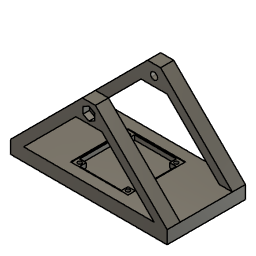
Pitch Control Base v3 (Autodesk Fusion 360 design; units mm, degrees)
Autodesk Fusion 360 part; units mm, degrees
note: some values were not read from the file. Set by a fixed rule: which sketch regions a step uses.
sketch "Sketch1" plane through (0, 0, 0) normal (0, 1, 0) x (1, 0, 0)
  line L0 (60, -30) -> (-60, -30)
  line L1 (-60, -30) -> (-60, 30)
  line L2 (-60, 30) -> (60, 30)
  line L3 (60, 30) -> (60, -30)
  line L4 (60, -30) -> (-60, 30) construction
  line L5 (-60, -30) -> (60, 30) construction
  constraint horizontal L0
  constraint perpendicular L0 L1
  constraint parallel L0 L2
  constraint parallel L1 L3
  constraint coincident L4 origin
  constraint coincident L5 origin
extrude "Extrude1" add sketch "Sketch1" along normal blind 10
sketch "Sketch2" plane through (0, 0, 0) normal (0, 0, 1) x (1, 0, 0)
  line L0 (-60, 10) -> (-5, 65)
  line L1 (-5, 65) -> (5, 65)
  line L2 (5, 65) -> (60, 10)
  line L3 (60, 10) -> (50, 10)
  line L4 (-50, 10) -> (-60, 10)
  line L5 (-50, 10) -> (-10, 50)
  line L6 (-10, 50) -> (10, 50)
  line L7 (10, 50) -> (50, 10)
  constraint horizontal L1
  constraint parallel L1 L3
  constraint horizontal L4
  constraint parallel L0 L5
  constraint parallel L4 L6
extrude "Extrude2" add sketch "Sketch2" along normal mid plane 60
sketch "Sketch3" plane through (0, 0, 30) normal (0, 0, 1) x (1, 0, 0)
  line L0 (50, 10) -> (-50, 10)
  line L1 (-50, 10) -> (-10, 50)
  line L2 (-10, 50) -> (10, 50)
  line L3 (10, 50) -> (50, 10)
  line L4 (60, 10) -> (5, 65)
  line L5 (5, 65) -> (-5, 65)
  line L6 (-5, 65) -> (-60, 10)
  line L7 (-60, 10) -> (-60, 0)
  line L8 (-60, 0) -> (60, 0)
  line L9 (60, 0) -> (60, 10)
  line L10 (0, 62) -> (4.5, 59.5)
  line L11 (4.5, 59.5) -> (4.5, 54.5)
  line L12 (4.5, 54.5) -> (0, 52)
  line L13 (0, 52) -> (-4.5, 54.5)
  line L14 (-4.5, 54.5) -> (-4.5, 59.5)
  line L15 (-4.5, 59.5) -> (0, 62)
  circle A0 centre (0, 57) radius 2.7
  dimension "d11" = 5.4
  constraint vertical L11
  constraint parallel L10 L13
  constraint parallel L11 L14
  constraint parallel L12 L15
  measures "d11" diameter of A0
extrude "Extrude3" cut sketch "Sketch3" against normal blind 5 contours L10 L11 L12 L13 L14 L15 | A0
sketch "Sketch4" plane through (0, 65, 0) normal (0, 1, 0) x (-1, 0, 0)
  line L0 (5, -30) -> (5, 30)
  line L1 (5, 30) -> (-5, 30)
  line L2 (-5, 30) -> (-5, -30)
  line L3 (-5, -30) -> (5, -30)
  line L4 (60, 20) -> (-60, 20)
  line L5 (-60, 20) -> (-60, -20)
  line L6 (-60, -20) -> (60, -20)
  line L7 (60, -20) -> (60, 20)
  line L8 (60, 20) -> (-60, -20) construction
  line L9 (-60, 20) -> (60, -20) construction
  dimension "d7" = 120
  dimension "d8" = 40
  constraint horizontal L4
  constraint perpendicular L4 L5
  constraint parallel L4 L6
  constraint parallel L5 L7
  constraint coincident L8 origin
  constraint coincident L9 origin
  measures "d7" distance of L5.end L6.end
  measures "d8" distance of L4.end L5.end
extrude "Extrude4" cut sketch "Sketch4" against normal blind 55 contours L0 L2 L4 L6 | L0 L4 L6 L7 | L2 L4 L5 L6
extrude "Extrude6" cut sketch "Sketch3" against normal blind 60 contours A0
sketch "Sketch6" plane through (0, 0, -30) normal (0, 0, -1) x (-1, 0, 0)
  circle A0 centre (0, 57) radius 2.7
  line L0 (-60, 10) -> (-60, 0)
  line L1 (-60, 0) -> (60, 0)
  line L2 (60, 0) -> (60, 10)
  line L3 (60, 10) -> (5, 65)
  line L4 (5, 65) -> (-5, 65)
  line L5 (-5, 65) -> (-60, 10)
  line L6 (-50, 10) -> (-10, 50)
  line L7 (-10, 50) -> (10, 50)
  line L8 (10, 50) -> (50, 10)
  line L9 (50, 10) -> (-50, 10)
  circle A1 centre (0, 57) radius 5
  dimension "d18" = 10
  constraint concentric A0 A1
  measures "d18" diameter of A1
extrude "Extrude7" cut sketch "Sketch6" against normal blind 3 contours A1
sketch "Sketch7" plane through (0, 10, 0) normal (0, 1, 0) x (-1, 0, 0)
  line L0 (50, 20) -> (50, 30)
  line L1 (50, 30) -> (-50, 30)
  line L2 (-50, 30) -> (-50, 20)
  line L3 (-50, 20) -> (-60, 20)
  line L4 (-60, 20) -> (-60, -20)
  line L5 (-60, -20) -> (-50, -20)
  line L6 (-50, -20) -> (-50, -30)
  line L7 (-50, -30) -> (50, -30)
  line L8 (50, -30) -> (50, -20)
  line L9 (50, -20) -> (60, -20)
  line L10 (60, -20) -> (60, 20)
  line L11 (60, 20) -> (50, 20)
  line L12 (21, -21) -> (-21, -21)
  line L13 (-21, -21) -> (-21, 21)
  line L14 (-21, 21) -> (21, 21)
  line L15 (21, 21) -> (21, -21)
  line L16 (21, -21) -> (-21, 21) construction
  line L17 (-21, -21) -> (21, 21) construction
  line L18 (-21, 21) -> (-16, 21)
  line L19 (-16, 21) -> (-16, 16)
  line L20 (-16, 16) -> (-21, 16)
  line L21 (-21, 16) -> (-21, 21)
  line L22 (-21, -21) -> (-16, -21)
  line L23 (-16, -21) -> (-16, -16)
  line L24 (-16, -16) -> (-21, -16)
  line L25 (-21, -16) -> (-21, -21)
  line L26 (21, 21) -> (16, 21)
  line L27 (16, 21) -> (16, 16)
  line L28 (16, 16) -> (21, 16)
  line L29 (21, 16) -> (21, 21)
  line L30 (21, -21) -> (16, -21)
  line L31 (16, -21) -> (16, -16)
  line L32 (16, -16) -> (21, -16)
  line L33 (21, -16) -> (21, -21)
  line L34 (22, -22) -> (-22, -22)
  line L35 (-22, -22) -> (-22, 22)
  line L36 (-22, 22) -> (22, 22)
  line L37 (22, 22) -> (22, -22)
  line L38 (22, -22) -> (-22, 22) construction
  line L39 (-22, -22) -> (22, 22) construction
  dimension "d21" = 42
  dimension "d22" = 42
  dimension "d23" = 5
  dimension "d24" = 5
  dimension "d25" = 5
  dimension "d26" = 5
  dimension "d27" = 5
  dimension "d28" = 5
  dimension "d29" = 5
  dimension "d30" = 5
  dimension "d33" = 44
  dimension "d34" = 44
  constraint horizontal L12
  constraint perpendicular L12 L13
  constraint parallel L12 L14
  constraint parallel L13 L15
  constraint coincident L16 origin
  constraint coincident L17 origin
  constraint horizontal L18
  constraint vertical L19
  constraint horizontal L20
  constraint vertical L21
  constraint horizontal L22
  constraint vertical L23
  constraint horizontal L24
  constraint vertical L25
  constraint horizontal L26
  constraint vertical L27
  constraint horizontal L28
  constraint vertical L29
  constraint horizontal L30
  constraint vertical L31
  constraint horizontal L32
  constraint vertical L33
  constraint horizontal L34
  constraint perpendicular L34 L35
  constraint parallel L34 L36
  constraint parallel L35 L37
  constraint coincident L38 origin
  constraint coincident L39 origin
  measures "d21" distance of L13.end L14.end
  measures "d22" distance of L12.end L13.end
  measures "d23" distance of L13.end L18.end
  measures "d24" distance of L13.end L20.end
  measures "d25" distance of L12.end L22.end
  measures "d26" distance of L12.end L24.end
  measures "d27" distance of L14.end L26.end
  measures "d28" distance of L14.end L28.end
  measures "d29" distance of L12.start L30.end
  measures "d30" distance of L12.start L32.end
  measures "d33" distance of L35.end L36.end
  measures "d34" distance of L34.end L35.end
extrude "Extrude8" cut sketch "Sketch7" against normal blind 4 contours L12 L13 L14 L15 L19 L20 L23 L24 L27 L28 L31 L32
extrude "Extrude9" cut sketch "Sketch7" against normal blind 0.5 contours L12 L15 L30 L31 L32 L33 | L12 L13 L22 L23 L24 L25 | L14 L15 L26 L27 L28 L29 | L13 L14 L18 L19 L20 L21 | L34 L35 L36 L37
sketch "Sketch8" plane through (0, 9.5, 0) normal (0, 1, 0) x (-1, 0, 0)
  line L0 (16, -16) -> (16, -21)
  line L1 (16, -21) -> (-16, -21)
  line L2 (-16, -21) -> (-16, -16)
  line L3 (-16, -16) -> (-21, -16)
  line L4 (-21, -16) -> (-21, 16)
  line L5 (-21, 16) -> (-16, 16)
  line L6 (-16, 16) -> (-16, 21)
  line L7 (-16, 21) -> (16, 21)
  line L8 (16, 21) -> (16, 16)
  line L9 (16, 16) -> (21, 16)
  line L10 (21, 16) -> (21, -16)
  line L11 (21, -16) -> (16, -16)
  line L12 (22, 22) -> (-22, 22)
  line L13 (-22, 22) -> (-22, -22)
  line L14 (-22, -22) -> (22, -22)
  line L15 (22, -22) -> (22, 22)
  circle A0 centre (-18.5, 18.5) radius 1.5
  circle A1 centre (18.5, 18.5) radius 1.5
  circle A2 centre (-18.5, -18.5) radius 1.5
  circle A3 centre (18.5, -18.5) radius 1.5
  dimension "d37" = 3
  dimension "d38" = 3
  dimension "d39" = 3
  dimension "d40" = 3
  measures "d37" diameter of A0
  measures "d38" diameter of A1
  measures "d39" diameter of A2
  measures "d40" diameter of A3
extrude "Extrude10" cut sketch "Sketch8" against normal blind 6 contours A0 | A1 | A2 | A3
